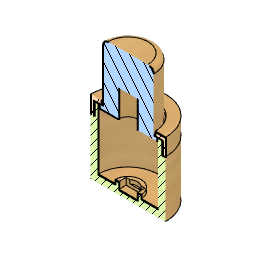
probatio_block_top_dual_pistons v16 (Autodesk Fusion 360 archive; units mm, degrees)
design "Button_Hall_2.0_Parametric"
Autodesk Fusion 360 part; units mm, degrees
sketch "Sketch1" plane through (0, 0, 0) normal (0, 1, 0) x (1, 0, 0) in component "Base"
  circle A0 centre (0, 0) radius 10
  dimension "d63" = 20
  constraint coincident A0.centre origin
  measures "d63" diameter of A0
extrude "Extrude1" add sketch "Sketch1" along normal blind 2 makes body 1 in component "Base"
sketch "Sketch2" plane through (0, 2, 0) normal (0, 1, 0) x (-1, 0, 0) in component "Base"
  circle A0 centre (0, 0) radius 10
  circle A1 centre (0, 0) radius 8
  dimension "d66" = -2
extrude "Extrude2" add sketch "Sketch2" along normal blind 13 bodies 1 in component "Base"
sketch "Sketch3" plane through (0, 15, 0) normal (0, 1, 0) x (-1, 0, 0) in component "Base"
  circle A0 centre (0, 0) radius 8
  circle A1 centre (0, 0) radius 10
  circle A2 centre (0, 0) radius 9
  dimension "d69" = 1
extrude "Extrude3" add sketch "Sketch3" along normal blind 3.5 contours A2 bodies 1 in component "Base"
sketch "Sketch2 (2)" plane through (0, 15, 0) normal (0, 1, 0) x (-1, 0, 0) in component "Ring"
  circle A0 centre (0, 0) radius 9 construction
  circle A1 centre (0, 0) radius 10
  circle A2 centre (0, 0) radius 9.2
  dimension "offset_bottom" = 0.2
extrude "Extrude1'" add sketch "Sketch2 (2)" along normal blind 3.5 separate body makes body 2 in component "Ring"
sketch "Sketch3 (2)" plane through (0, 18.5, 0) normal (0, 1, 0) x (-1, 0, 0) in component "Ring"
  circle A0 centre (0, 0) radius 9.2 construction
  circle A1 centre (0, 0) radius 10
extrude "Extrude2'" add sketch "Sketch3 (2)" along normal blind 1 bodies 2 in component "Ring"
sketch "Sketch4" plane through (0, 19.5, 0) normal (0, 1, 0) x (-1, 0, 0) in component "Ring"
  circle A0 centre (0, 0) radius 10
  circle A1 centre (0, 0) radius 9
  circle A2 centre (0, 0) radius 7.2
  dimension "d77" = 18
  dimension "diameter_apperture" = 14.4
  constraint coincident A0.centre A1.centre
  constraint concentric A1 A2
  measures "d77" diameter of A1
  measures "diameter_apperture" diameter of A2
extrude "Extrude3'" cut sketch "Sketch4" against normal blind 1 contours A2 bodies 2 in component "Ring"
sketch "Sketch1 (2)" plane through (0, 18.5, 0) normal (0, -1, 0) x (1, 0, 0) in component "Top"
  circle A0 centre (0, 0) radius 7.2 construction
  circle A1 centre (0, 0) radius 9.2 construction
  circle A2 centre (0, 0) radius 7.7
  dimension "diameter_bottom_disc" = 15.4
  constraint concentric A0 A2
  measures "diameter_bottom_disc" diameter of A2
extrude "Extrude1''" add sketch "Sketch1 (2)" along normal blind 1 separate body makes body 3 in component "Top"
ref_plane "WorkPlane2" through (0, 17.1186, 0) normal (0, 0, 1) x (-1, 0, 0)
sketch "Sketch2 (3)" plane through (0, 18.5, 0) normal (0, 1, 0) x (-1, 0, 0) in component "Top"
  circle A0 centre (0, 0) radius 7.7
  circle A1 centre (0, 0) radius 6.8
  dimension "diameter_tower" = 13.6
  constraint concentric A0 A1
  measures "diameter_tower" diameter of A1
extrude "Extrude2''" add sketch "Sketch2 (3)" along normal blind 15.5 contours A1 bodies 3 in component "Top"
sketch "Sketch3 (3)" plane through (0, 17.5, 0) normal (0, -1, 0) x (1, 0, 0) in component "Top"
  circle A0 centre (0, 0) radius 7.7
  circle A1 centre (0, 0) radius 2.5
  dimension "d90" = 5
  constraint coincident A0.centre A1.centre
  measures "d90" diameter of A1
extrude "Extrude3''" cut sketch "Sketch3 (3)" against normal blind 7.2 contours A1 bodies 3 in component "Top"
sketch "Sketch4 (2)" plane through (0, 2, 0) normal (0, 1, 0) x (-1, 0, 0) in component "Base"
  circle A0 centre (0, 0) radius 8
  circle A1 centre (0, 0) radius 2.5
  circle A2 centre (0, 0) radius 3.5
  dimension "d98" = 5
  dimension "d99" = 1
  constraint concentric A0 A1
  measures "d98" diameter of A1
extrude "Extrude4" add sketch "Sketch4 (2)" along normal blind 1 contours A2 bodies 1 in component "Base"
ref_plane "WorkPlane1" through (0, 2.8235, -3.5) normal (0, 0, -1) x (1, 0, 0) in component "Base"
ref_plane "WorkPlane2" through (0, 2.5, 3.5) normal (0, 0, 1) x (1, 0, 0) in component "Base"
ref_plane "WorkPlane3" through (0, 2.8235, 0) normal (0, 0, -1) x (1, 0, 0) in component "Base"
sketch "Sketch6" plane through (0, 2.8235, 0) normal (0, 0, -1) x (1, 0, 0) in component "Base"
  line L0 (-3.5, -0.1765) -> (3.5, -0.1765)
  line L1 (-10, 2.8235) -> (10, 2.8235)
  line L2 (3.5, 0.8235) -> (-3.5, 0.8235) construction
  line L3 (-3.5, -0.1765) -> (-3.5, 0.8235) construction
  line L4 (3.5, -0.1765) -> (3.5, 0.8235) construction
  line L5 (-3.5, -0.1765) -> (-2.5, -0.1765) construction
  line L6 (-2.5, -0.1765) -> (-2.5, 0.8235) construction
  line L7 (-2.5, 0.8235) -> (-3.5, 0.8235) construction
  line L8 (-3.5, 0.8235) -> (-3.5, -0.1765) construction
  line L9 (3.5, -0.1765) -> (2.5, -0.1765) construction
  line L10 (2.5, -0.1765) -> (2.5, 0.8235) construction
  line L11 (2.5, 0.8235) -> (3.5, 0.8235) construction
  line L12 (3.5, 0.8235) -> (3.5, -0.1765) construction
  line L13 (-2.5, -0.1765) -> (2.5, -0.1765)
  line L14 (2.5, -0.1765) -> (2.5, 1.6235)
  line L15 (2.5, 1.6235) -> (-2.5, 1.6235)
  line L16 (-2.5, 1.6235) -> (-2.5, -0.1765)
  dimension "d104" = 1
  dimension "d105" = 1
  dimension "d106" = 1
  dimension "d107" = 1
  dimension "d108" = 1.8
  constraint coincident L0.start L3.start
  constraint coincident L2.end L3.end
  constraint coincident L0.end L4.start
  constraint coincident L2.start L4.end
  constraint horizontal L5
  constraint vertical L6
  constraint horizontal L7
  constraint vertical L8
  constraint horizontal L9
  constraint vertical L10
  constraint horizontal L11
  constraint vertical L12
  constraint perpendicular L13 L14
  constraint parallel L13 L15
  constraint parallel L14 L16
  measures "d104" distance of L0.start L2.end
  measures "d105" distance of L0.start L5.end
  measures "d106" distance of L0.end L9.end
  measures "d107" distance of L0.end L2.start
  measures "d108" distance of L5.end L15.end
extrude "Extrude5" cut sketch "Sketch6" along normal blind 2 bodies 1 in component "Base"
extrude "Extrude6" cut sketch "Sketch6" against normal through all bodies 1 in component "Base"
ref_plane "WorkPlane4" through (0, 2.8235, 2) normal (0, 0, -1) x (1, 0, 0) in component "Base"
sketch "Sketch7" plane through (0, 2.8235, 2) normal (0, 0, -1) x (1, 0, 0) in component "Base"
  line L0 (2.5, -0.1765) -> (2.5, 1.6235)
  line L1 (-2.5, -0.1765) -> (2.5, -0.1765)
  line L2 (2.5, 1.6235) -> (-2.5, 1.6235)
  line L3 (-2.5, 1.6235) -> (-2.5, -0.1765)
extrude "Extrude7" cut sketch "Sketch7" against normal through all draft 5 bodies 1 in component "Base"
fillet "Fillet1" radius 1.5 1 edges at (6.3398, 34, -2.459) on bodies 3 in component "Top"
component "Base" placed x (1, 0, 0) y (0, 1, 0) z (0, 0, 1) at (0, 0, 0)
component "Ring" placed x (1, 0, 0) y (0, 1, 0) z (0, 0, 1) at (0, 0, 0)
component "Top" placed x (1, 0, 0) y (0, 1, 0) z (0, 0, 1) at (0, 0, 0)
equation "base_diameter = 20 mm"
equation "tolerance = 0.2 mm"
equation "wall_thickness = 1 mm"
equation "base_total_height = 18.5 mm"
equation "base_ring_height = 3.5 mm"
equation "base_bottom_thickness = 2 mm"
equation "d63 = base_diameter"
equation "d64 = base_bottom_thickness"
equation "d66 = -2 * wall_thickness"
equation "d67 = base_total_height - base_bottom_thickness - base_ring_height"
equation "d69 = wall_thickness"
equation "d70 = base_ring_height"
equation "offset_bottom = tolerance"
equation "d73 = base_ring_height"
equation "d75 = wall_thickness"
equation "d77 = base_diameter - 2 * wall_thickness"
equation "diameter_apperture = base_diameter - 6 * wall_thickness + 2 * tolerance"
equation "d79 = -wall_thickness"
equation "diameter_bottom_disc = base_diameter - 4 * wall_thickness - 3 * tolerance"
equation "d83 = wall_thickness"
equation "diameter_tower = base_diameter - 6 * wall_thickness - 2 * tolerance"
equation "top_safety_margin = 1 mm" comment "To avoid the top to get stuck inside base"
equation "d88 = base_total_height - 2 * wall_thickness - base_bottom_thickness + top_safety_margin"
equation "d90 = magnet_diameter"
equation "magnet_diameter = 5 mm"
equation "magnet_height = 2.4 mm"
equation "magnet_quantity = 3"
equation "d95 = -magnet_height * magnet_quantity"
equation "spring_diameter = 5 mm"
equation "d98 = spring_diameter"
equation "d99 = wall_thickness"
equation "d100 = wall_thickness"
equation "d104 = wall_thickness"
equation "d105 = wall_thickness"
equation "d106 = wall_thickness"
equation "d107 = wall_thickness"
